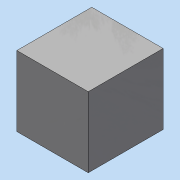
# Autodesk Inventor part: BLANK-BC-10002
Saved by Autodesk Inventor 2016 (Build 200138000, 138)
## iProperties
Created: 2015-12-02
Part Number: BLANK-BC-10002
Project: DIPOLO BC-3T- SIRIUS
Cost Center: 1504002005
Material: Aço Carbono
Document SubType Name: Modeling
Designer: reinaldo.basilo
Mass: 14747.8 g
Surface Area: 912.32 cm^2
Volume: 1873.92 cm^3
Density: 7.87 g/cm^3
Appearance: Steel
Description: Base de fechamento magnético dos blocos central.
RuleStatus: InUse
AfterMaterialChange0: file://_iMaterial
AfterAnyiPropertyChange0: file://_iMaterial
AfterDocNew0: file://_Naming_par
AfterDocNew1: file://_NameStart
AfterDocNew2: file://_NameStart1
AfterDocNew3: file://_Materiais
DocNumber: XXXXX-XXX-XXXX-00-001.ipt
Folder: .
Title: DIPOLO BC-3T- SIRIUS
Author: Reinaldo.Basílio
Subject: BLANK-BC-10002
Autodesk Inventor part; units mm, degrees
ref_plane "YZ Plane" through (0, 0, 0) normal (1, 0, 0) x (0, 1, 0)
ref_plane "XZ Plane" through (0, 0, 0) normal (0, 1, 0) x (-1, 0, 0)
ref_plane "XY Plane" through (0, 0, 0) normal (0, 0, 1) x (1, 0, 0)
sketch "Sketch5" plane through (0, 0, 0) normal (0, 1, 0) x (-1, 0, 0)
  line L0 (64, 60) -> (-64, 60)
  line L1 (-64, 60) -> (-64, -60)
  line L2 (-64, -60) -> (64, -60)
  line L3 (64, -60) -> (64, 60)
  point P0 (0, 0)
  point P1 (64, 0)
  point P2 (0, 60)
  dimension "d8" = 128
  dimension "d9" = 120
  constraints: 8 end point, 2 midpoint, 2 parallel, 1 horizontal, 1 horizontal alignment, 1 perpendicular, 1 vertical alignment
  measures "d8" distance of L0.start L0.end
  measures "d9" distance of L0.end L1.end
extrude "Extrusion5" add sketch "Sketch5" along normal blind 122
sketch "Sketch6" plane through (-64, 0, -60) normal (-1, 0, 0) x (0, 0, 1)
  line L0 (0, 0) -> (120, 0)
  line L1 (120, 0) -> (120, 122)
  line L2 (0, 0) -> (120, 0)
  line L3 (120, 0) -> (120, 120)
  line L4 (120, 120) -> (0, 120)
  line L5 (0, 120) -> (0, 0)
  line L6 (0, 0) -> (120, 0) projected
  line L7 (120, 0) -> (120, 122) projected
  line L8 (0, 122) -> (120, 122) projected
  line L9 (0, 0) -> (0, 122) projected
  point P0 (447.5, 0)
  dimension "d12" = 120
  constraints: 12 end point, 2 parallel, 1 collinear, 1 horizontal, 1 perpendicular
  measures "d12" distance between parallel lines of L0 L4
extrude "Extrusion6" [suppressed]
chamfer "Chamfer1" [suppressed]
body "Solid5"
